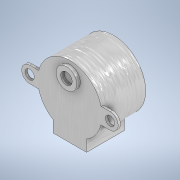
# Autodesk Inventor part: Шаговый мотор
Saved by Autodesk Inventor 2023 (Build 270158000, 158)
## iProperties
Created: 2022-10-09
Part Number: Шаговый мотор
Material: Типовые
Document SubType Name: Modeling
Designer: Admin
Density: 1 g/cm^3
Appearance: По умолчанию
Author: Admin
Autodesk Inventor part; units mm, degrees
ref_plane "YZ Plane" through (0, 0, 0) normal (1, 0, 0) x (0, 1, 0)
ref_plane "XZ Plane" through (0, 0, 0) normal (0, 1, 0) x (-1, 0, 0)
ref_plane "XY Plane" through (0, 0, 0) normal (0, 0, 1) x (1, 0, 0)
sketch "Эскиз1" plane through (0, 0, 0) normal (0, 0, 1) x (1, 0, 0)
  circle A0 centre (0, 0) radius 14
  circle A1 centre (-17.5, 0) radius 2
  circle A2 centre (17.5, 0) radius 2
  circle A3 centre (0, 8) radius 4.5
  circle A4 centre (0, 8) radius 2.5
  line L0 (-7.25, -11.9765) -> (-7.25, -17)
  line L1 (-7.25, -17) -> (7.25, -17)
  line L2 (7.25, -17) -> (7.25, -11.9765)
  circle A5 centre (-17.5, 0) radius 3.5
  circle A6 centre (17.5, 0) radius 3.5
  line L3 (-17.5, 3.5) -> (-13.5554, 3.5)
  line L4 (-17.5, -3.5) -> (-13.5554, -3.5)
  line L5 (17.5, 3.5) -> (13.5554, 3.5)
  line L6 (17.5, -3.5) -> (13.5554, -3.5)
  line L7 (0, 0) -> (0, 3.849) construction
  line L8 (-2, 9.5) -> (2, 9.5)
  line L9 (2, 6.5) -> (-2, 6.5)
  line L10 (0, 8) -> (-1.0582, 8) construction
  point P0 (0, -17)
  dimension "d0" = 35
  dimension "d1" = 17
  dimension "d2" = 8
  dimension "d4" = 7
  dimension "d5" = 4
  dimension "d6" = 9
  dimension "d7" = 5
  dimension "d8" = 3
  dimension "d9" = 28
  dimension "d10" = 14.5
  dimension "d19" = 3.9446
  constraints: 22 end point, 14 point on circle, 7 centre point, 4 coincident, 4 point on line, 3 horizontal, 3 horizontal alignment, 2 parallel, 2 perpendicular, 2 tangent, 2 vertical, 2 vertical alignment, 1 equal radius, 1 midpoint, 1 symmetric about line, 1 other
  measures "d0" distance of A1.centre A2.centre
  measures "d1" distance from line of A2.centre L1
  measures "d2" distance of A3.centre point (0, 0)
  measures "d4" distance between parallel lines of L6 L5
  measures "d5" diameter of A1
  measures "d6" diameter of A3
  measures "d7" diameter of A4
  measures "d8" distance between parallel lines of L9 L8
  measures "d9" diameter of A0
  measures "d10" distance between parallel lines of L0 L2
  measures "d19" distance of L5.start L5.end
extrude "Выдавливание1" add sketch "Эскиз1" against normal blind 19 contours A0 | A3 | A4 L9 L8 | L8 A4 | A4 L9
extrude "Выдавливание2" add sketch "Эскиз1" against normal blind 1 contours A6 L6 A0 | A0 L5 A6 | A6 | A0 A5 L3 | A5 | A0 L4 A5
extrude "Выдавливание3" add sketch "Эскиз1" against normal blind 16.5 contours L2 L1 L0 A0
extrude "Выдавливание4" add sketch "Эскиз1" along normal blind 1.5 contours A3
